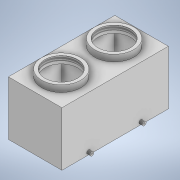
# Autodesk Inventor part: BoxChem
Saved by Autodesk Inventor 2022 (Build 260153070, 153G)
## iProperties
Created: 2021-07-20
Part Number: BoxChem
Material: Generic
Document SubType Name: Modeling
Designer: Eakawit_kor
Density: 1 g/cm^3
Appearance: Default
Author: Eakawit_kor
Autodesk Inventor part; units mm, degrees
ref_plane "YZ Plane" through (0, 0, 0) normal (1, 0, 0) x (0, 1, 0)
ref_plane "XZ Plane" through (0, 0, 0) normal (0, 1, 0) x (-1, 0, 0)
ref_plane "XY Plane" through (0, 0, 0) normal (0, 0, 1) x (1, 0, 0)
sketch "Sketch1" plane through (0, 0, 0) normal (0, 0, 1) x (1, 0, 0)
  line L0 (0, 0) -> (82, 0)
  line L1 (82, 0) -> (82, 82)
  line L2 (82, 82) -> (0, 82)
  line L3 (0, 82) -> (0, 0)
  dimension "d0" = 82
  dimension "d1" = 82
  constraints: 8 end point, 2 parallel, 1 horizontal, 1 perpendicular
  measures "d0" distance of L2.end L0.start
  measures "d1" distance of L1.end L2.end
extrude "Extrusion1" add sketch "Sketch1" along normal blind 163
shell "Shell1" thickness 1 removed faces 1 at (54.6667, 82, 54.3333)
sketch "Sketch6" plane through (82, 0, 0) normal (1, 0, 0) x (0, 0, -1)
  circle A0 centre (-122, 4) radius 1
  circle A1 centre (-122, 4) radius 3
  line L0 (0, 0) -> (0, 82) projected
  line L1 (0, 0) -> (-163, 0) projected
  line L2 (-163, 0) -> (-163, 82) projected
  dimension "d18" = 2
  dimension "d19" = 2
  dimension "d21" = 4
  dimension "d50" = 41
  constraints: 2 centre point
  measures "d18" diameter of A0
  measures "d19" radial gap between concentric circles of A1 A0
  measures "d21" distance from line of L1 A0.centre
  measures "d50" distance from line of A0.centre L2
extrude "Extrusion5" add sketch "Sketch6" along normal blind 5
thread "Thread1" size "M6x1" class "6g" standard "ANSI Metric M Profile" length 7.15
sketch "Sketch7" plane through (82, 4, 122) normal (1, 0, 0) x (0, 0, -1)
  circle A0 centre (0, 0) radius 1 projected
  circle A1 centre (0, 0) radius 1
  point P0 (122, -4)
  constraints: 1 centre point, 1 coincident
extrude "Extrusion6" cut sketch "Sketch7" against normal blind 5
sketch "Sketch8" plane through (0, 82, 0) normal (0, 1, 0) x (1, 0, 0)
  line L0 (0, 0) -> (0, -163) projected
  line L1 (82, 0) -> (82, -163) projected
  line L2 (0, 0) -> (82, 0)
  line L3 (82, 0) -> (82, -163)
  line L4 (82, -163) -> (0, -163)
  line L5 (0, -163) -> (0, 0)
  point P0 (0, -163)
  constraints: 8 end point, 2 parallel, 1 horizontal, 1 perpendicular
extrude "Extrusion7" add sketch "Sketch8" along normal blind 1
sketch "Sketch9" plane through (0, 83, 0) normal (0, 1, 0) x (1, 0, 0)
  circle A0 centre (40, -122) radius 25
  circle A1 centre (40, -122) radius 30
  line L0 (0, 0) -> (0, -163) projected
  line L1 (0, -163) -> (82, -163) projected
  line L2 (1, -1) -> (1, -162) projected
  line L3 (1, -81.5) -> (81, -81.5)
  line L4 (81, -1) -> (81, -162) projected
  dimension "d30" = 50
  dimension "d31" = 40
  dimension "d32" = 41
  dimension "d33" = 5
  constraints: 2 centre point, 2 end point, 2 midpoint
  measures "d30" diameter of A0
  measures "d31" distance from line of L0 A0.centre
  measures "d32" distance from line of L1 A0.centre
  measures "d33" radial gap between concentric circles of A1 A0
extrude "Extrusion8" add sketch "Sketch9" along normal blind 10
sketch "Sketch10" plane through (40, 83, 122) normal (0, 1, 0) x (1, 0, 0)
  circle A0 centre (0, 0) radius 25
  point P0 (-40, 122)
  constraints: 1 centre point
extrude "Extrusion9" cut sketch "Sketch10" against normal blind 10
thread "Thread2" size "M50x4" class "6H" standard "ANSI Metric M Profile" length 7.15
sketch "Sketch12" plane through (1, 1, 1) normal (0, 1, 0) x (1, 0, 0)
  line L0 (0, 0) -> (0, -161) projected
  line L1 (0, -81) -> (80, -81)
  line L2 (80, -81) -> (80, -80)
  line L3 (80, -80) -> (0, -80)
  line L4 (0, -80) -> (0, -81)
  line L5 (80, 0) -> (80, -161) projected
  line L6 (0, -161) -> (80, -161) projected
  point P0 (-1, 1)
  point P1 (0, -80)
  dimension "d44" = 1
  dimension "d45" = 80
  constraints: 8 end point, 2 parallel, 1 collinear, 1 horizontal, 1 perpendicular, 1 point on line
  measures "d44" distance between parallel lines of L1 L3
  measures "d45" distance between parallel lines of L6 L1
extrude "Extrusion11" add sketch "Sketch12" along normal blind 80 contours L3 L2 L1 L0
sketch "Sketch3" plane through (1, 82, 1) normal (0, 0, 1) x (1, 0, 0)
  line L0 (0, -81) -> (80, -81)
  line L1 (80, -81) -> (0, -78)
  line L2 (0, -78) -> (0, -81)
  point P0 (-1, -82)
  dimension "d5" = 3
  constraints: 6 end point, 1 perpendicular
  measures "d5" distance of L1.end L0.start
extrude "Extrusion12" add sketch "Sketch3" along normal up to surface (161 mm away)
pattern_linear "Rectangular Pattern1" count 2 spacing 81 along (0, 0, -1) of "Extrusion8", "Extrusion9"
pattern_linear "Rectangular Pattern3" count 2 spacing 80 along (0, 0, -1) of "Extrusion5", "Extrusion6"
body "Solid1"
